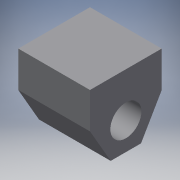
# Autodesk Inventor part: Linear Stage
Saved by Autodesk Inventor 2016 (Build 200138000, 138)
## iProperties
Created: 2014-03-13
Part Number: Linear Stage
Material: Generic
Document SubType Name: Modeling
Designer: John
Density: 1 g/cm^3
Appearance: Default
Author: John
Autodesk Inventor part; units mm, degrees
ref_plane "YZ Plane" through (0, 0, 0) normal (1, 0, 0) x (0, 1, 0)
ref_plane "XZ Plane" through (0, 0, 0) normal (0, 1, 0) x (-1, 0, 0)
ref_plane "XY Plane" through (0, 0, 0) normal (0, 0, 1) x (1, 0, 0)
sketch "Sketch1" plane through (0, 0, 0) normal (1, 0, 0) x (0, 1, 0)
  line L0 (0, 0) -> (19.05, 0)
  line L1 (19.05, 0) -> (19.05, -19.05)
  line L2 (19.05, -19.05) -> (0, -19.05)
  line L3 (0, -19.05) -> (0, 0)
  circle A0 centre (7.3025, -9.525) radius 4.1275
  line L4 (0, -9.525) -> (7.3025, -9.525) construction
  line L5 (9.525, 0) -> (0, -5.4993)
  line L6 (9.525, -19.05) -> (0, -13.5507)
  dimension "d0" = 19.05
  dimension "d1" = 19.05
  dimension "d2" = 8.255
  dimension "d3" = 3.175
  dimension "d4" = 30
  constraints: 14 end point, 3 midpoint, 2 parallel, 2 perpendicular, 2 point on line, 1 centre point, 1 horizontal, 1 other
  measures "d0" distance of L1.end L2.end
  measures "d1" distance of L0.end L1.end
  measures "d2" diameter of A0
  measures "d3" distance edge to line of A0 L3
  measures "d4" angle of L0 L5
extrude "Extrusion1" add sketch "Sketch1" along normal blind 19.05 contours L0 L1 L2 L6 L3 L5
body "Solid1"
